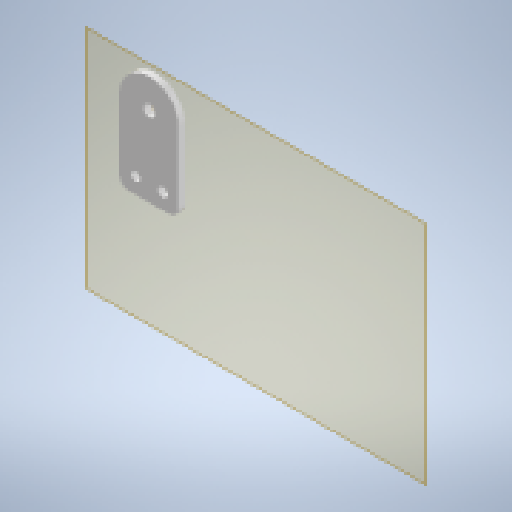
# Autodesk Inventor part: Soporte Motor2
Saved by Autodesk Inventor 2023 (Build 270158000, 158)
## iProperties
Created: 2023-04-22
Part Number: Soporte Motor2
Material: Genérico
Document SubType Name: Modeling
Designer: sergi
Density: 1 g/cm^3
Appearance: Valor por defecto
Author: sergi
Autodesk Inventor part; units mm, degrees
ref_plane "YZ Plane" through (0, 0, 0) normal (1, 0, 0) x (0, 1, 0)
ref_plane "XZ Plane" through (0, 0, 0) normal (0, 1, 0) x (-1, 0, 0)
ref_plane "XY Plane" through (0, 0, 0) normal (0, 0, 1) x (1, 0, 0)
ref_plane "Plano de trabajo1" through (0, 0, 0) normal (0, 0, 1) x (1, 0, 0)
sketch "Boceto1" plane through (0, 0, 0) normal (0, 0, 1) x (1, 0, 0)
  arc A0 (23.25, 32) -> (26.25, 35) centre (23.25, 35) ccw projected
  line L0 (23.25, 32) -> (10.75, 32) projected
  arc A1 (7.75, 35) -> (10.75, 32) centre (10.75, 35) ccw projected
  line L1 (7.75, 35) -> (7.75, 57) projected
  arc A2 (26.25, 57) -> (7.75, 57) centre (17, 57) ccw projected
  line L2 (26.25, 57) -> (26.25, 35) projected
  circle A3 centre (12.75, 37) radius 2.5 projected
  circle A4 centre (21.25, 37) radius 2.5 projected
  circle A5 centre (17, 57) radius 8.5 projected
  arc A6 (15.882, 58) -> (18.118, 58) centre (17, 57) ccw projected
  circle A7 centre (17, 57) radius 1.75
  circle A8 centre (12.75, 37) radius 1.5
  circle A9 centre (21.25, 37) radius 1.5
  point P0 (0, 0)
  dimension "d0" = 3.5
  dimension "d1" = 3
  dimension "d2" = 3
  constraints: 3 centre point, 3 coincident
  measures "d0" diameter of A7
  measures "d1" diameter of A8
  measures "d2" diameter of A9
extrude "Extrusión1" add sketch "Boceto1" along normal blind 2 contours L0 A1 L1 A2 L2 A0 | A3 | A4 | A5
sketch "Boceto2" plane through (0, 0, 0) normal (0, 0, -1) x (-1, 0, 0)
  circle A0 centre (-17, 57) radius 1.75 projected
  circle A1 centre (-17, 57) radius 2.5
  point P0 (0, 0)
  dimension "d5" = 5
  constraints: 1 centre point, 1 coincident
  measures "d5" diameter of A1
extrude "Extrusión2" add sketch "Boceto2" along normal blind 2
fillet "Empalme1" radius 2 1 edges at (19.5, 57, 0)
